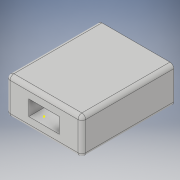
# Autodesk Inventor part: USB Plug Protector v2
Saved by Autodesk Inventor 2019 (Build 230136000, 136)
## iProperties
Created: 2021-08-13
Part Number: USB Plug Protector v2
Material: Generic
Document SubType Name: Modeling
Designer: Lix
Density: 1 g/cm^3
Appearance: Default
Author: Lix
Autodesk Inventor part; units mm, degrees
ref_plane "YZ Plane" through (0, 0, 0) normal (1, 0, 0) x (0, 1, 0)
ref_plane "XZ Plane" through (0, 0, 0) normal (0, 1, 0) x (-1, 0, 0)
ref_plane "XY Plane" through (0, 0, 0) normal (0, 0, 1) x (1, 0, 0)
sketch "Sketch1" plane through (0, 0, 0) normal (0, 0, 1) x (1, 0, 0)
  line L0 (-17.75, 0) -> (17.75, 0) construction
  line L1 (0, 8) -> (0, -8) construction
  line L2 (-6.5, 3.6221) -> (6.5, 3.6221)
  line L3 (6.5, 3.6221) -> (6.5, -3.6221)
  line L4 (6.5, -3.6221) -> (-6.5, -3.6221)
  line L5 (-6.5, -3.6221) -> (-6.5, 3.6221)
  line L6 (-6.5, 3.6221) -> (6.5, -3.6221) construction
  line L7 (6.5, 3.6221) -> (-6.5, -3.6221) construction
  line L8 (-17.75, 7.5) -> (17.75, 7.5)
  line L9 (17.75, 7.5) -> (17.75, -7.5)
  line L10 (17.75, -7.5) -> (-17.75, -7.5)
  line L11 (-17.75, -7.5) -> (-17.75, 7.5)
  line L12 (-17.75, 7.5) -> (17.75, -7.5) construction
  line L13 (17.75, 7.5) -> (-17.75, -7.5) construction
  line L14 (19.75, 9.5) -> (-19.75, 9.5)
  line L15 (-19.75, 9.5) -> (-19.75, -9.5)
  line L16 (-19.75, -9.5) -> (19.75, -9.5)
  line L17 (19.75, -9.5) -> (19.75, 9.5)
  point P0 (0, 0)
  point P1 (0, 0)
  dimension "d0" = 35.5
  dimension "d2" = 16
  dimension "d3" = 13
  dimension "d8" = 35.5
  dimension "d9" = 15
  dimension "d10" = 2
  constraints: 36 end point, 6 midpoint, 6 parallel, 3 horizontal, 3 perpendicular, 1 coincident, 1 vertical, 3 other
  measures "d0" distance of L0.start L0.end
  measures "d2" distance of L1.start L1.end
  measures "d3" distance of L3.end L4.end
  measures "d8" distance of L9.end L10.end
  measures "d9" distance of L8.end L9.end
  measures "d10" distance between parallel lines of L8 L14
sketch "Sketch2" plane through (0, 0, 0) normal (0, 0, 1) x (1, 0, 0)
  circle A0 centre (16.2358, 0.0652) radius 1.2658
  circle A1 centre (-16.2297, 0.0693) radius 2.6113
  circle A2 centre (-16.2209, 0.071) radius 1.2886
  circle A3 centre (16.2226, 0.0693) radius 2.6113
  circle A4 centre (9.0155, -3.0732) radius 4.1082
  circle A5 centre (-9.0155, -3.0529) radius 4.1296
  line L0 (17.2205, -0.737) -> (11.7242, -6.1827)
  line L1 (-9.6279, -7.1374) -> (9.6209, -7.1374)
  line L2 (-11.7313, -6.1827) -> (-17.2276, -0.737)
  line L3 (-17.2276, 0.879) -> (-11.7313, 6.3247)
  line L4 (11.7242, 6.3247) -> (17.2205, 0.879)
  line L5 (-9.6279, 7.2795) -> (9.6209, 7.2795)
  circle A6 centre (8.9431, 3.0732) radius 4.2681
  circle A7 centre (-8.9501, 3.0732) radius 4.2681
  line L6 (-9.0155, 3.0732) -> (9.0155, -3.0732)
  point P0 (0, 0)
  point P1 (-0.0035, 8.5079)
  point P2 (0, 0)
  constraints: 14 end point, 8 centre point, 1 midpoint
extrude "Extrusion1" add sketch "Sketch1" along normal blind 20 contours L17 L16 L15 L14
sketch "Sketch3" plane through (0, 0, 20) normal (0, 0, 1) x (1, 0, 0)
  line L0 (-8, 4) -> (8, 4)
  line L1 (8, 4) -> (8, -4)
  line L2 (8, -4) -> (-8, -4)
  line L3 (-8, -4) -> (-8, 4)
  line L4 (-8, 4) -> (8, -4) construction
  line L5 (8, 4) -> (-8, -4) construction
  line L6 (17.75, 7.5) -> (17.75, -7.5) projected
  line L7 (17.75, -7.5) -> (-17.75, -7.5) projected
  line L8 (-17.75, -7.5) -> (-17.75, 7.5) projected
  line L9 (-17.75, 7.5) -> (17.75, 7.5) projected
  line L10 (19.75, 9.5) -> (-19.75, 9.5) projected
  line L11 (-19.75, 9.5) -> (-19.75, -9.5) projected
  line L12 (-19.75, -9.5) -> (19.75, -9.5) projected
  line L13 (19.75, -9.5) -> (19.75, 9.5) projected
  point P0 (0, 0)
  dimension "d13" = 16
  dimension "d14" = 8
  constraints: 12 end point, 2 midpoint, 2 parallel, 1 horizontal, 1 perpendicular
  measures "d13" distance of L1.end L2.end
  measures "d14" distance of L0.end L1.end
extrude "Extrusion2" add sketch "Sketch3" along normal blind 28 contours L6 L7 L8 L9 | L13 L12 L11 L10
sketch "Sketch4" plane through (0, 0, 48) normal (0, 0, 1) x (1, 0, 0)
  point P0 (0, 0)
fillet "Fillet1" radius 2 8 edges at (19.75, 9.5, 24) (19.75, -9.5, 24) (-19.75, -9.5, 24) (-19.75, 9.5, 24) (-19.75, 0, 48) (0, 9.5, 48) (0, -9.5, 48) (19.75, 0, 48)
body "Solid1"
